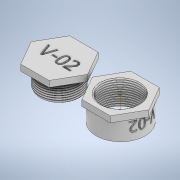
# Autodesk Inventor part: boltAndNut1_625x12-V02
Saved by Autodesk Inventor 2021.1 (Build 251245000, 245)
## iProperties
Created: 2020-08-22
Part Number: boltAndNut1_625x12-V02
Material: Generic
Document SubType Name: Modeling
Designer: robst
Density: 1 g/cm^3
Appearance: Default
Author: robst
Autodesk Inventor part; units mm, degrees
ref_plane "XZ Plane" through (0, 0, 0) normal (0, 1, 0) x (-1, 0, 0)
ref_plane "XY Plane" through (0, 0, 0) normal (0, 0, 1) x (1, 0, 0)
sketch "Sketch4" plane through (0, 0, 0) normal (0, 1, 0) x (-1, 0, 0)
  circle A0 centre (0, 0) radius 25.4
  circle A1 centre (0, 0) radius 19.7206
  dimension "d4" = 50.8
  dimension "d5" = 39.4411
  constraints: 2 centre point, 2 coincident
  measures "d4" diameter of A0
  measures "d5" diameter of A1
extrude "NutShaft" add sketch "Sketch4" against normal blind 25.4
sketch "Sketch6" plane through (0, 0, 0) normal (0, 0, 1) x (1, 0, 0)
  line L0 (19.7206, -25.4) -> (19.7206, 0) projected
  line L1 (19.7206, 2.1167) -> (20.8305, 2.7575)
  line L2 (20.8305, 2.9555) -> (19.7206, 3.5963)
  line L3 (19.7206, 3.5963) -> (19.7206, 2.1167)
  line L4 (0, -31.1993) -> (0, 9.3956) projected
  arc A0 (20.8305, 2.7575) -> (20.8305, 2.9555) centre (20.7734, 2.8565) ccw
  point P0 (0, 0)
  dimension "d33" = 60
  dimension "d35" = 0.1143
  dimension "d36" = 20.8877
  dimension "d37" = 2.1167
  constraints: 6 end point, 2 point on circle, 2 tangent, 1 centre point, 1 collinear, 1 equal length, 1 vertical
  measures "d33" angle of L1 L2
  measures "d35" radius of A0
  measures "d37" distance of L1.start L0.end
coil "CoilForNut" sketch "Sketch6" operation cut axis through (0, -10, 0) along (0, -1, 0) pitch 2.1167 turns 14 hand right
sketch "Sketch7" plane through (0, 0, 0) normal (0, 1, 0) x (-1, 0, 0)
  line L0 (0, 0) -> (63.5, 0) construction
  line L1 (34.1706, 0) -> (48.8353, 25.4)
  line L2 (48.8353, 25.4) -> (78.1647, 25.4)
  line L3 (78.1647, 25.4) -> (92.8294, 0)
  line L4 (92.8294, 0) -> (78.1647, -25.4)
  line L5 (78.1647, -25.4) -> (48.8353, -25.4)
  line L6 (48.8353, -25.4) -> (34.1706, 0)
  dimension "d46" = 63.5
  dimension "d50" = 50.8
  constraints: 14 end point, 2 horizontal, 1 coincident, 13 other
  measures "d46" distance of L0.start L0.end
  measures "d50" distance between parallel lines of L2 L5
extrude "BoltHexHead" add sketch "Sketch7" against normal blind 6.35
sketch "Sketch8" plane through (0, -6.35, 0) normal (0, -1, 0) x (1, 0, 0)
  line L0 (-48.8353, 25.4) -> (-78.1647, 25.4) projected
  line L1 (-34.1706, 0) -> (-48.8353, 25.4) projected
  line L2 (-48.8353, -25.4) -> (-34.1706, 0) projected
  line L3 (-78.1647, -25.4) -> (-48.8353, -25.4) projected
  line L4 (-92.8294, 0) -> (-78.1647, -25.4) projected
  line L5 (-78.1647, 25.4) -> (-92.8294, 0) projected
  line L6 (-78.1647, 25.4) -> (-69.0759, -25.4) construction
  line L7 (-48.8353, 25.4) -> (-78.1647, -25.4) construction
  circle A0 centre (-63.5, 0) radius 20.4699
  point P0 (0, 0)
  dimension "d49" = 40.9397
  constraints: 4 end point, 1 centre point, 1 midpoint, 1 parallel, 1 point on line
  measures "d49" diameter of A0
extrude "BoltShaft" add sketch "Sketch8" along normal blind 19.05 contours A0
sketch "Sketch9" plane through (0, 0, 0) normal (0, 0, 1) x (1, 0, 0)
  line L0 (-43.0301, -6.35) -> (-43.0301, -25.4) projected
  line L1 (-83.9699, -25.4) -> (-43.0301, -25.4) projected
  line L2 (-43.0301, -27.5167) -> (-44.3116, -28.2565)
  line L3 (-44.3116, -28.5821) -> (-43.0301, -29.3219)
  line L4 (-43.0301, -29.3219) -> (-43.0301, -27.5167)
  line L5 (-63.5, -25.4) -> (-63.5, 0) construction
  line L6 (-78.1647, 0) -> (-48.8353, 0) construction
  arc A0 (-44.3116, -28.2565) -> (-44.3116, -28.5821) centre (-44.2176, -28.4193) ccw
  point P0 (0, 0)
  dimension "d53" = 60
  dimension "d54" = 0.188
  dimension "d56" = 20.4699
  dimension "d57" = 19.0944
  dimension "d66" = 2.1167
  constraints: 8 end point, 2 midpoint, 2 point on circle, 2 tangent, 1 centre point, 1 equal length
  measures "d53" angle of L2 L3
  measures "d54" radius of A0
  measures "d56" distance between parallel lines of L4 L5
  measures "d57" distance edge to line of A0 L5
  measures "d66" distance of L2.start L0.end
coil "CoilForBolt" sketch "Sketch9" operation cut axis through (-63.5, -25.4, 0) along (0, 1, 0) pitch 2.1167 turns 12 hand right
sketch "Sketch11" plane through (0, 0, 0) normal (0, 1, 0) x (1, 0, 0)
  line L0 (-78.1647, -25.4) -> (-92.8294, 0) construction
  line L1 (-48.8353, 25.4) -> (-34.1706, 0) construction
  line L2 (-92.8294, 0) -> (-34.1706, 0) construction
  line L3 (-70.9152, 6.35) -> (-75.2892, -6.35)
  line L4 (-75.2892, -6.35) -> (-77.1108, -6.35)
  line L5 (-77.1108, -6.35) -> (-81.4848, 6.35)
  line L6 (-81.4848, 6.35) -> (-79.6735, 6.35)
  line L7 (-79.6735, 6.35) -> (-76.1537, -4.199)
  line L8 (-76.1537, -4.199) -> (-72.6339, 6.35)
  line L9 (-72.6339, 6.35) -> (-70.9152, 6.35)
  line L10 (-65.265, -1.5643) -> (-70.0713, -1.5643)
  line L11 (-70.0713, -1.5643) -> (-70.0713, -0.0206)
  line L12 (-70.0713, -0.0206) -> (-65.265, -0.0206)
  line L13 (-65.265, -0.0206) -> (-65.265, -1.5643)
  spline S0 degree 2 poles (-55.6731, 0) (-55.6731, -3.4169) (-57.6594, -6.6176) (-59.7281, -6.6176) knots 0 0 0 1 2 2 2
  spline S1 degree 2 poles (-59.7281, -6.6176) (-61.8276, -6.6176) (-63.7933, -3.3551) (-63.7933, -0.0103) knots 0 0 0 1 2 2 2
  spline S2 degree 2 poles (-63.7933, -0.0103) (-63.7933, 3.4271) (-61.807, 6.6073) (-59.7281, 6.6073) knots 0 0 0 1 2 2 2
  spline S3 degree 2 poles (-59.7281, 6.6073) (-57.6389, 6.6073) (-55.6731, 3.3139) (-55.6731, 0) knots 0 0 0 1 2 2 2
  spline S4 degree 2 poles (-57.855, -3.8697) (-57.608, -3.2419) (-57.4021, -1.3071) (-57.4021, 0) knots 0 0 0 1 2 2 2
  spline S5 degree 2 poles (-57.4021, 0) (-57.4021, 1.3071) (-57.608, 3.2316) (-57.8653, 3.88) knots 0 0 0 1 2 2 2
  spline S6 degree 2 poles (-57.8653, 3.88) (-58.1226, 4.5284) (-59.0179, 5.1973) (-59.7281, 5.1973) knots 0 0 0 1 2 2 2
  spline S7 degree 2 poles (-59.7281, 5.1973) (-60.4382, 5.1973) (-61.3542, 4.5284) (-61.6218, 3.8594) knots 0 0 0 1 2 2 2
  spline S8 degree 2 poles (-61.6218, 3.8594) (-61.8791, 3.211) (-62.0643, 1.235) (-62.0643, -0.0103) knots 0 0 0 1 2 2 2
  spline S9 degree 2 poles (-62.0643, -0.0103) (-62.0643, -1.3482) (-61.8996, -3.139) (-61.632, -3.8388) knots 0 0 0 1 2 2 2
  spline S10 degree 2 poles (-61.632, -3.8388) (-61.385, -4.4975) (-60.4691, -5.2076) (-59.7281, -5.2076) knots 0 0 0 1 2 2 2
  spline S11 degree 2 poles (-59.7281, -5.2076) (-59.0282, -5.2076) (-58.1123, -4.5387) (-57.855, -3.8697) knots 0 0 0 1 2 2 2
  line L14 (-46.215, -6.35) -> (-54.047, -6.35)
  line L15 (-54.047, -6.35) -> (-54.047, -4.5489)
  spline S12 degree 2 poles (-54.047, -4.5489) (-53.2031, -3.7565) (-51.7005, -2.2848) (-50.9801, -1.4923) knots 0 0 0 1 2 2 2
  spline S13 degree 2 poles (-50.9801, -1.4923) (-49.529, 0.1029) (-48.4689, 2.0172) (-48.4689, 3.0361) knots 0 0 0 1 2 2 2
  spline S14 degree 2 poles (-48.4689, 3.0361) (-48.4689, 3.5712) (-48.7983, 4.374) (-49.0967, 4.6313) knots 0 0 0 1 2 2 2
  spline S15 degree 2 poles (-49.0967, 4.6313) (-49.3952, 4.8886) (-50.1774, 5.1459) (-50.6508, 5.1459) knots 0 0 0 1 2 2 2
  spline S16 degree 2 poles (-50.6508, 5.1459) (-51.1036, 5.1459) (-52.0299, 4.9194) (-52.4518, 4.7445) knots 0 0 0 1 2 2 2
  spline S17 degree 2 poles (-52.4518, 4.7445) (-52.812, 4.6004) (-53.481, 4.1887) (-53.6868, 4.0447) knots 0 0 0 1 2 2 2
  line L16 (-53.6868, 4.0447) -> (-53.7795, 4.0447)
  line L17 (-53.7795, 4.0447) -> (-53.7795, 5.856)
  spline S18 degree 2 poles (-53.7795, 5.856) (-53.2546, 6.1133) (-51.3712, 6.6176) (-50.5273, 6.6176) knots 0 0 0 1 2 2 2
  spline S19 degree 2 poles (-50.5273, 6.6176) (-48.7468, 6.6176) (-46.7399, 4.7342) (-46.7399, 3.1287) knots 0 0 0 1 2 2 2
  spline S20 degree 2 poles (-46.7399, 3.1287) (-46.7399, 2.3774) (-47.0898, 1.1218) (-47.3986, 0.5866) knots 0 0 0 1 2 2 2
  spline S21 degree 2 poles (-47.3986, 0.5866) (-47.7073, 0.0309) (-48.6027, -1.06) (-49.0967, -1.5849) knots 0 0 0 1 2 2 2
  spline S22 degree 2 poles (-49.0967, -1.5849) (-49.8995, -2.4597) (-51.8652, -4.3328) (-52.4518, -4.8783) knots 0 0 0 1 2 2 2
  line L18 (-52.4518, -4.8783) -> (-46.215, -4.8783)
  line L19 (-46.215, -4.8783) -> (-46.215, -6.35)
  point P0 (0, 0)
  constraints: 2 end point, 2 horizontal
extrude "EmbossForBolt" cut sketch "Sketch11" against normal blind 2.54
ref_plane "Work Plane4" through (25.4, 0, 0) normal (1, 0, 0) x (0, 1, 0)
sketch "Sketch12" plane through (25.4, 0, 0) normal (1, 0, 0) x (0, 1, 0)
  line L0 (0, 25.4) -> (-25.4, 25.4)
  line L1 (0, -25.4) -> (0, 25.4)
  line L2 (0, -25.4) -> (-25.4, -25.4)
  line L3 (-25.4, 25.4) -> (-25.4, -25.4) projected
  line L4 (-12.7, 25.4) -> (-12.7, -25.4) construction
  line L5 (-17.78, -5.9322) -> (-7.62, -9.4313)
  line L6 (-7.62, -9.4313) -> (-7.62, -10.8887)
  line L7 (-7.62, -10.8887) -> (-17.78, -14.3878)
  line L8 (-17.78, -14.3878) -> (-17.78, -12.9388)
  line L9 (-17.78, -12.9388) -> (-9.3408, -10.1229)
  line L10 (-9.3408, -10.1229) -> (-17.78, -7.3071)
  line L11 (-17.78, -7.3071) -> (-17.78, -5.9322)
  line L12 (-11.4485, -1.412) -> (-11.4485, -5.257)
  line L13 (-11.4485, -5.257) -> (-12.6835, -5.257)
  line L14 (-12.6835, -5.257) -> (-12.6835, -1.412)
  line L15 (-12.6835, -1.412) -> (-11.4485, -1.412)
  spline S0 degree 2 poles (-12.7, 6.2615) (-9.9665, 6.2615) (-7.4059, 4.6724) (-7.4059, 3.0175) knots 0 0 0 1 2 2 2
  spline S1 degree 2 poles (-7.4059, 3.0175) (-7.4059, 1.3379) (-10.0159, -0.2347) (-12.6918, -0.2347) knots 0 0 0 1 2 2 2
  spline S2 degree 2 poles (-12.6918, -0.2347) (-15.4417, -0.2347) (-17.9858, 1.3544) (-17.9858, 3.0175) knots 0 0 0 1 2 2 2
  spline S3 degree 2 poles (-17.9858, 3.0175) (-17.9858, 4.6889) (-15.3512, 6.2615) (-12.7, 6.2615) knots 0 0 0 1 2 2 2
  spline S4 degree 2 poles (-9.6042, 4.516) (-10.1065, 4.7136) (-11.6544, 4.8783) (-12.7, 4.8783) knots 0 0 0 1 2 2 2
  spline S5 degree 2 poles (-12.7, 4.8783) (-13.7456, 4.8783) (-15.2853, 4.7136) (-15.804, 4.5078) knots 0 0 0 1 2 2 2
  spline S6 degree 2 poles (-15.804, 4.5078) (-16.3227, 4.3019) (-16.8579, 3.5856) (-16.8579, 3.0175) knots 0 0 0 1 2 2 2
  spline S7 degree 2 poles (-16.8579, 3.0175) (-16.8579, 2.4494) (-16.3227, 1.7167) (-15.7875, 1.5026) knots 0 0 0 1 2 2 2
  spline S8 degree 2 poles (-15.7875, 1.5026) (-15.2688, 1.2968) (-13.688, 1.1486) (-12.6918, 1.1486) knots 0 0 0 1 2 2 2
  spline S9 degree 2 poles (-12.6918, 1.1486) (-11.6214, 1.1486) (-10.1888, 1.2803) (-9.6289, 1.4944) knots 0 0 0 1 2 2 2
  spline S10 degree 2 poles (-9.6289, 1.4944) (-9.102, 1.692) (-8.5339, 2.4247) (-8.5339, 3.0175) knots 0 0 0 1 2 2 2
  spline S11 degree 2 poles (-8.5339, 3.0175) (-8.5339, 3.5774) (-9.0691, 4.3102) (-9.6042, 4.516) knots 0 0 0 1 2 2 2
  line L16 (-7.62, 13.828) -> (-7.62, 7.5624)
  line L17 (-7.62, 7.5624) -> (-9.0608, 7.5624)
  spline S12 degree 2 poles (-9.0608, 7.5624) (-9.6948, 8.2375) (-10.8722, 9.4396) (-11.5062, 10.0159) knots 0 0 0 1 2 2 2
  spline S13 degree 2 poles (-11.5062, 10.0159) (-12.7823, 11.1768) (-14.3137, 12.0249) (-15.1288, 12.0249) knots 0 0 0 1 2 2 2
  spline S14 degree 2 poles (-15.1288, 12.0249) (-15.557, 12.0249) (-16.1992, 11.7614) (-16.405, 11.5226) knots 0 0 0 1 2 2 2
  spline S15 degree 2 poles (-16.405, 11.5226) (-16.6109, 11.2839) (-16.8167, 10.6581) (-16.8167, 10.2794) knots 0 0 0 1 2 2 2
  spline S16 degree 2 poles (-16.8167, 10.2794) (-16.8167, 9.9171) (-16.6356, 9.1761) (-16.4956, 8.8385) knots 0 0 0 1 2 2 2
  spline S17 degree 2 poles (-16.4956, 8.8385) (-16.3803, 8.5504) (-16.051, 8.0152) (-15.9357, 7.8505) knots 0 0 0 1 2 2 2
  line L18 (-15.9357, 7.8505) -> (-15.9357, 7.7764)
  line L19 (-15.9357, 7.7764) -> (-17.3848, 7.7764)
  spline S18 degree 2 poles (-17.3848, 7.7764) (-17.5906, 8.1963) (-17.9941, 9.703) (-17.9941, 10.3782) knots 0 0 0 1 2 2 2
  spline S19 degree 2 poles (-17.9941, 10.3782) (-17.9941, 11.8026) (-16.4874, 13.4081) (-15.2029, 13.4081) knots 0 0 0 1 2 2 2
  spline S20 degree 2 poles (-15.2029, 13.4081) (-14.6019, 13.4081) (-13.5974, 13.1281) (-13.1693, 12.8811) knots 0 0 0 1 2 2 2
  spline S21 degree 2 poles (-13.1693, 12.8811) (-12.7247, 12.6341) (-11.852, 11.9178) (-11.4321, 11.5226) knots 0 0 0 1 2 2 2
  spline S22 degree 2 poles (-11.4321, 11.5226) (-10.7322, 10.8804) (-9.2337, 9.3078) (-8.7974, 8.8385) knots 0 0 0 1 2 2 2
  line L20 (-8.7974, 8.8385) -> (-8.7974, 13.828)
  line L21 (-8.7974, 13.828) -> (-7.62, 13.828)
  point P0 (0, 0)
  constraints: 8 end point, 2 midpoint, 1 coincident, 1 vertical
emboss "EmbossForNut" sketch "Sketch12" operation cut depth 2.54 direction (-1, 0, 0) wrap yes faces at (-25.3176, -16.9333, -2.0439) contours L5 L6 L7 L8 L9 L10 L11 | L12 L13 L14 L15 | S0 S1 S2 S3 | L16 L17 S12 S13 S14 S15 S16 S17 L18 L19 S18 S19 S20 S21 S22 L20 L21
sketch "Sketch13" plane through (0, 0, 0) normal (0, 1, 0) x (1, 0, 0)
  line L0 (29.3294, 0) -> (14.6647, -25.4)
  line L1 (14.6647, -25.4) -> (-14.6647, -25.4)
  line L2 (-14.6647, -25.4) -> (-29.3294, 0)
  line L3 (-29.3294, 0) -> (-14.6647, 25.4)
  line L4 (-14.6647, 25.4) -> (14.6647, 25.4)
  line L5 (14.6647, 25.4) -> (29.3294, 0)
  line L6 (19.9576, 11.1478) -> (22.1751, 12.3864) projected
  circle A0 centre (0, 0) radius 22.86
  dimension "d73" = 50.8
  constraints: 12 end point, 2 coincident, 1 horizontal, 16 other
  measures "d73" distance between parallel lines of L1 L4
extrude "NutHexHead" add sketch "Sketch13" against normal blind 6.35
sketch "Sketch14" plane through (0, -25.4, 0) normal (0, -1, 0) x (1, 0, 0)
  line L0 (-34.1706, 0) -> (-48.8353, 25.4) projected
  line L1 (-48.8353, -25.4) -> (-34.1706, 0) projected
  line L2 (-78.1647, -25.4) -> (-48.8353, -25.4) projected
  line L3 (-92.8294, 0) -> (-78.1647, -25.4) projected
  line L4 (-78.1647, 25.4) -> (-92.8294, 0) projected
  line L5 (-48.8353, 25.4) -> (-78.1647, 25.4) projected
  line L6 (-48.8353, 25.4) -> (-78.1647, -25.4) construction
  line L7 (-92.8294, 0) -> (-78.1647, 25.4) construction
  line L8 (-48.8353, -25.4) -> (-78.1647, 25.4) construction
  circle A0 centre (-63.5, 0) radius 12.7
  point P0 (0, 0)
  constraints: 4 end point, 1 centre point, 1 midpoint
extrude "HoleForBolt" cut sketch "Sketch14" against normal blind 19.05 contours A0
equation "\"d4\" = nutOutsideDiameter"
equation "\"d5\" = b2MinorDiameterMax"
equation "\"d35\" = b2RootRadius"
equation "\"d36\" = 0.5 * b2MajorDiameterMax"
equation "\"d37\" = pitch"
equation "\"d38\" = pitch"
equation "\"d39\" = cuttingLengthOfNut"
equation "\"d49\" = a2MajorDiameterMin"
equation "\"d54\" = a2RootRadius"
equation "\"d56\" = 0.5 * a2MajorDiameterMin"
equation "\"d57\" = 0.5 * a2MinorDiameterMin"
equation "\"d66\" = pitch"
equation "\"d58\" = pitch"
equation "\"b2ThreadDepthMin\" = 0.91694"
equation "\"a2MajorDiameterMax\" = 41.22928"
equation "\"a2MajorDiameterMin\" = 40.93972"
equation "\"a2PitchDiameterMax\" = 39.85514"
equation "\"a2PitchDiamterMin\" = 39.70528"
equation "\"a2MinorDiameterMax\" = 38.7096"
equation "\"a2MinorDiameterMin\" = 38.1889"
equation "\"a2CrestFlatMax\" = 0.4318"
equation "\"a2CrestFlatMin\" = 0.1778"
equation "\"a2RootFlatMax\" = 0.38862"
equation "\"a2RootFlatMin\" = 0.26416"
equation "\"a2RootRadiusMax\" = 0.22352"
equation "\"a2RootRadiusMin\" = 0.1524"
equation "\"a2ThreadDepthMax\" = 1.52146"
equation "\"a2ThreadDepthMin\" = 1.11506"
equation "\"b2MajorDiameterMax\" = 41.77538"
equation "\"b2MajorDiameterMin\" = 41.275"
equation "\"b2PitchDiameterMax\" = 40.09644"
equation "\"b2PitchDiameterMin\" = 39.90086"
equation "\"b2MinorDiameterMax\" = 39.44112"
equation "\"b2MinorDiameterMin\" = 38.98392"
equation "\"b2CrestFlatMax\" = 7.9502"
equation "\"b2CrestFlatMin\" = 0.41656"
equation "\"b2RootFlatMax\" = 0.26416"
equation "\"b2RootFlatMin\" = 0.0889"
equation "\"b2RootRadiusMax\" = 0.1524"
equation "\"b2RootRadiusMin\" = 0.0762"
equation "\"b2ThreadDepthMax\" = 1.397"
equation "\"b2MajorDiameter\" = 0.5 * b2MajorDiameterMin + 0.5 * b2MajorDiameterMax"
equation "\"b2MinorDiameter\" = 0.5 * b2MinorDiameterMin + 0.5 * b2MinorDiameterMax"
equation "\"b2RootRadius\" = 0.5 * b2RootRadiusMin + 0.5 * b2RootRadiusMax"
equation "\"a2MajorDiameter\" = 0.5 * a2MajorDiameterMin + 0.5 * a2MajorDiameterMax"
equation "\"a2MinorDiameter\" = 0.5 * a2MinorDiameterMin + 0.5 * a2MinorDiameterMax"
equation "\"a2RootRadius\" = 0.5 * a2RootRadiusMin + 0.5 * a2RootRadiusMax"
equation "\"nutOutsideDiameter\" = 50.8"
equation "\"d70\" = 0.5 * nutOutsideDiameter"
equation "\"heightOfNut\" = 25.4"
equation "\"pitch\" = 2.116667"
equation "\"cuttingLengthOfNut\" = 29.633333"
body "Solid2"
